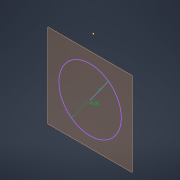
# Autodesk Inventor part: Clemm
Saved by Autodesk Inventor 2022 (Build 260153070, 153G)
## iProperties
Created: 2021-11-19
Part Number: Clemm
Material: Типовые
Document SubType Name: Modeling
Designer: kalugin_a
Density: 1 g/cm^3
Appearance: По умолчанию
Author: kalugin_a
Autodesk Inventor part; units mm, degrees
ref_plane "YZ Plane" through (0, 0, 0) normal (1, 0, 0) x (0, 1, 0)
ref_plane "XZ Plane" through (0, 0, 0) normal (0, 1, 0) x (-1, 0, 0)
ref_plane "XY Plane" through (0, 0, 0) normal (0, 0, 1) x (1, 0, 0)
sketch "Эскиз4" plane through (0, 0, 0) normal (0, 0, 1) x (1, 0, 0)
  line L0 (1, -3.5) -> (-1, -3.5)
  line L1 (-2.5, -2) -> (-2.5, 2)
  line L2 (-1, 3.5) -> (1, 3.5)
  line L3 (2.5, 2) -> (2.5, -2)
  line L4 (2.5, -3.5) -> (-2.5, 3.5) construction
  line L5 (-2.5, -3.5) -> (2.5, 3.5) construction
  arc A0 (2.5, 2) -> (1, 3.5) centre (1, 2) ccw
  arc A1 (-1, 3.5) -> (-2.5, 2) centre (-1, 2) ccw
  arc A2 (-2.5, -2) -> (-1, -3.5) centre (-1, -2) ccw
  arc A3 (1, -3.5) -> (2.5, -2) centre (1, -2) ccw
  point P0 (0, 0)
  point P1 (0, -3)
  point P2 (0, 3)
  dimension "d15" = 5
  dimension "d16" = 7
  dimension "d17" = 1.5
  dimension "d18" = 1.5
  constraints: 12 end point, 8 point on circle, 8 point on line, 8 tangent, 4 centre point, 2 equal radius, 2 midpoint, 2 parallel, 1 horizontal, 1 perpendicular
  measures "d15" distance of L4.end L5.end
  measures "d16" distance of L5.start L4.end
  measures "d17" radius of A0
  measures "d18" radius of A1
extrude "Выдавливание2" add sketch "Эскиз4" along normal blind 10
